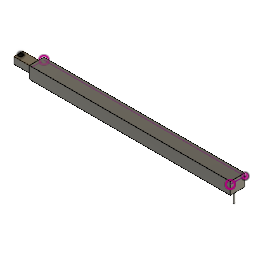
Outer Tie Rod (Autodesk Fusion 360 design; units mm, degrees)
Autodesk Fusion 360 part; units mm, degrees
sketch "Sketch1" plane through (0, 0, 0) normal (0, 0, 1) x (1, 0, 0)
  line L0 (0, 0) -> (165, 0)
  line L1 (165, 0) -> (165, -12)
  line L2 (165, -12) -> (0, -12)
  line L3 (0, -12) -> (0, 0)
  circle A0 centre (162.2, -6) radius 0.8
  dimension "d16" = 165
  dimension "d17" = 12
  dimension "d57" = 1.6
  dimension "d58" = 2.8
  dimension "d59" = 6
  constraint horizontal L0
  constraint vertical L1
  constraint horizontal L2
  constraint vertical L3
  constraint coincident L0.start L3.end
  measures "d16" distance of L0.start L0.end
  measures "d17" distance of L0.start L2.end
  measures "d57" diameter of A0
  measures "d58" distance of L1 A0.centre
  measures "d59" distance of L0 A0.centre
extrude "Extrude7" add sketch "Sketch1" against normal blind 10 contours A0 makes body 1
extrude "Extrude1" add sketch "Sketch1" along normal blind 10 separate body contours L0 L1 L2 L3 | A0 makes body 2
sketch "Sketch3" plane through (0, 0, 0) normal (-1, 0, 0) x (0, -1, 0)
  line L0 (0, 0) -> (12, 0)
  line L1 (12, 0) -> (12, 10)
  line L2 (12, 10) -> (0, 10)
  line L3 (0, 10) -> (0, 0)
  line L4 (2.2, 7.8) -> (9.8, 7.8)
  line L5 (9.8, 7.8) -> (9.8, 2.2)
  line L6 (9.8, 2.2) -> (2.2, 2.2)
  line L7 (2.2, 2.2) -> (2.2, 7.8)
  dimension "d22" = 7.6
  dimension "d23" = 5.6
  dimension "d26" = 2.2
  dimension "d27" = 2.2
  constraint horizontal L4
  constraint vertical L5
  constraint horizontal L6
  constraint vertical L7
  measures "d22" distance of L4.start L4.end
  measures "d23" distance of L4.start L6.end
  measures "d26" distance of L3 L7
  measures "d27" distance of L2 L4
extrude "Extrude2" add sketch "Sketch3" along normal blind 15 contours L4 L5 L6 L7 bodies 2
sketch "Sketch5" plane through (0, 0, 7.8) normal (0, 0, 1) x (-1, 0, 0)
  line L0 (0, 2.2) -> (15, 2.2)
  line L1 (15, 2.2) -> (15, 9.8)
  line L2 (15, 9.8) -> (0, 9.8)
  line L3 (-165, 12) -> (-165, 0)
  line L4 (-165, 0) -> (0, 0)
  line L5 (0, 9.8) -> (0, 2.2)
  circle A0 centre (13, 6) radius 1.5
  dimension "d48" = 3
  dimension "d49" = 2
  dimension "d50" = 3.8
  measures "d48" diameter of A0
  measures "d49" distance of L1 A0.centre
  measures "d50" distance of L0 A0.centre
extrude "Extrude6" cut sketch "Sketch5" against normal blind 100 contours A0 bodies 2
equation "main_length = 165 mm"
equation "height = 10 mm"
equation "dowel_edge_width = 7.6 mm"
equation "dowel_edge_length = 15 mm"
equation "length = 180 mm"
equation "edge_hole_radius = 1.5 mm"
equation "dowel_edge_hole_small_distance = dowel_edge_width / 2"
equation "width = 12 mm"
equation "dowel_edge_height = 5.6 mm"
equation "d16 = main_length"
equation "d17 = width"
equation "d18 = height"
equation "dowel_edge_small_distance = ( width - dowel_edge_width ) / 2"
equation "dowel_edge_big_distance = ( height - dowel_edge_height ) / 2"
equation "d22 = dowel_edge_width"
equation "d23 = dowel_edge_height"
equation "d24 = dowel_edge_length"
equation "d26 = dowel_edge_big_distance"
equation "d27 = dowel_edge_small_distance"
equation "extra = 100 mm"
equation "dowel_edge_hole_secondary_distance = 2 mm"
equation "d48 = edge_hole_radius * 2"
equation "d49 = dowel_edge_hole_secondary_distance"
equation "d50 = dowel_edge_hole_small_distance"
equation "d51 = -extra"
equation "bearing_dowel_radius = 0.8 mm"
equation "bearing_dowel_length = 10 mm"
equation "bearing_dowel_big_distance = 2 mm + bearing_dowel_radius"
equation "bearing_dowel_small_distance = width / 2"
equation "d57 = bearing_dowel_radius * 2"
equation "d58 = bearing_dowel_big_distance"
equation "d59 = bearing_dowel_small_distance"
equation "d60 = -bearing_dowel_length"
